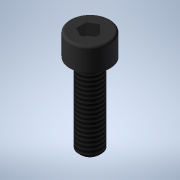
# Autodesk Inventor part: 62311400GA_2
Saved by Autodesk Inventor 2021 (Build 250183000, 183)
## iProperties
Created: 2026-04-27
Part Number: 62311400GA_2
Material: Generic
Catalog Web Link: www.3dfindit.com
Description: schr_typ_ga_geschl-Screws, Shaft Collars, Clamp Collars, Single-Split - Type GA, Diameter 10mm - 50mm, Material steel burnished and stainless steel 1.4305
Vendor: MAEDLER
Document SubType Name: Modeling
Designer: psAdmin
Manufacturer: MAEDLER
Mass: 0.312467 g
Surface Area: 3.54399 cm^2
Volume: 0.312467 cm^3
Density: 1 g/cm^3
Appearance: PSOLRGB-176-176-176
Category: PARTsolutions
Company: MAEDLER
Title: 62311400GA
Author: Cadenas PARTsolutions
Comments: Screws, Shaft Collars, Clamp Collars, Single-Split - Type GA, Diameter 10mm - 50mm, Material steel burnished and stainless steel 1.4305
PSOL_IDENT_0: {$CADENAS_DATA/23d-libs/maedler/antriebselemente/klemmringe_stellringe/klemmringe/geschl_klemmringe_
PSOL_IDENT_1: ausf_ga/schr_typ_ga_geschl.prj},176 {VTYP=3D},{NB=62311400GA_2},{LINA=62311400GA},{NN=schr_typ_ga_ge
PSOL_IDENT_2: schl},{DATE=10.04.2024 10:23:09},{GEOMDATE=07.01.2024 09:35:20},{VERSION=},{LINEID=2560},{WBVAR=},{W
PSOL_IDENT_3: BNUMERIC=}  {NB=62311400GA_2},{LINA=62311400GA},{KT=DUMMY},{ARTNR=62311400GA},{WEBSHOP=Produktdetail
PSOL_IDENT_4: s / Katalogseite / Montageanleitung},{MATK=Stahl},{MAT=Stahl C45 brüniert, Schraube mit Festigkeit 1
PSOL_IDENT_5: 2.9},{D4=4},{D3=3.24},{DK=7.0},{K=4},{SL=14},{SW=3.0},{SWT=2.0},{L=10},{V=0.4},{TN=schraube_typ_ga_s
PSOL_IDENT_6: t_14},{CTN=84839089}
NB: 62311400GA_2
NN: schr_typ_ga_geschl
NT: Screws, Shaft Collars, Clamp Collars, Single-Split - Type GA, Diameter 10mm - 50mm, Material steel burnished and stainless steel 1.4305
NBSYN: $ARTNR._2
LINA: 62311400GA
CATALOG: MÄDLER
ARTNR: 62311400GA
WEBSHOP: Produktdetails / Katalogseite / Montageanleitung
MATK: Stahl
MAT: Stahl C45 brüniert, Schraube mit Festigkeit 12.9
D4: 4
D3: 3.24
DK: 7
K: 4
SL: 14
SW: 3
SWT: 2
L: 10
V: 0.4
TN: schraube_typ_ga_st_14
CTN: 84839089
SUPPLIER: MAEDLER
ARTICLENO: 62311400GA_2
BOMINFO: 62311400GA
CREATOR: CADENAS GmbH
Autodesk Inventor part; units mm, degrees
sketch "Skizze_1" plane through (0, 0, 0) normal (0, 0, 1) x (1, 0, 0)
  line L0 (0, 18) -> (0, 0)
  line L1 (0, 0) -> (-1.5705, 0)
  line L2 (-1.5705, 0) -> (-2, 0.4295)
  line L3 (-2, 0.4295) -> (-2, 14)
  line L4 (-2, 14) -> (-3.5, 14)
  line L5 (-3.5, 14) -> (-3.5, 17.6)
  arc A0 (-3.1, 18) -> (-3.5, 17.6) centre (-3.1, 17.6) ccw
  line L6 (-3.1, 18) -> (0, 18)
  line L7 (0, 18) -> (0, 0)
  constraints: 16 end point, 2 point on circle, 1 centre point
revolve "Revolution1" add sketch "Skizze_1" angle 360 about axis through (0, 18, 0) along (0, 1, 0)
thread "Thread1" size "M4x0.7" class "6g" standard "ISO Metric profile" length 12.7132
sketch "Skizze_2" plane through (0, 18, 0) normal (0, 1, 0) x (-1, 0, 0)
  line L0 (-1.5, -0.866) -> (0, -1.7321)
  line L1 (0, -1.7321) -> (1.5, -0.866)
  line L2 (1.5, -0.866) -> (1.5, 0.866)
  line L3 (1.5, 0.866) -> (0, 1.7321)
  line L4 (0, 1.7321) -> (-1.5, 0.866)
  line L5 (-1.5, 0.866) -> (-1.5, -0.866)
  constraints: 12 end point
extrude "Extrusion1" cut sketch "Skizze_2" against normal blind 2
ref_plane "anf_ge_1_XY" through (0, 14, 0) normal (0, 1, 0) x (1, 0, 0)
ref_plane "anf_ge_1_YZ" through (0, 14, 0) normal (1, 0, 0) x (0, 0, -1)
ref_plane "anf_ge_1_ZX" through (0, 14, 0) normal (0, 0, -1) x (0, 1, 0)
body "Solid1"
